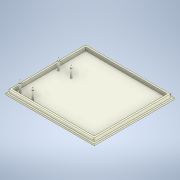
# Autodesk Inventor part: BARB_bottom
Saved by Autodesk Inventor 2022.3 (Build 263350000, 350)
## iProperties
Created: 2022-06-21
Part Number: BARB_bottom
Material: ABS Plastic
Document SubType Name: Modeling
Designer: abmos
Density: 1.06 g/cm^3
Appearance: Smooth - Ivory
Author: abmos
Autodesk Inventor part; units mm, degrees
ref_plane "YZ Plane" through (0, 0, 0) normal (1, 0, 0) x (0, 1, 0)
ref_plane "XZ Plane" through (0, 0, 0) normal (0, 1, 0) x (-1, 0, 0)
ref_plane "XY Plane" through (0, 0, 0) normal (0, 0, 1) x (1, 0, 0)
sketch "Master_XZ" plane through (0, 0, 0) normal (0, 1, 0) x (-1, 0, 0)
  line L0 (52.5, 47.5) -> (-52.5, 47.5)
  line L1 (-52.5, 47.5) -> (-52.5, -47.5)
  line L2 (-52.5, -47.5) -> (52.5, -47.5)
  line L3 (52.5, -47.5) -> (52.5, 47.5)
  line L4 (52.5, 47.5) -> (-52.5, -47.5) construction
  line L5 (-52.5, 47.5) -> (52.5, -47.5) construction
  line L6 (50.5, 45.5) -> (-50.5, 45.5)
  line L7 (-50.5, 45.5) -> (-50.5, -45.5)
  line L8 (-50.5, -45.5) -> (50.5, -45.5)
  line L9 (50.5, -45.5) -> (50.5, 45.5)
  line L10 (48.5, 43.5) -> (-48.5, 43.5)
  line L11 (-48.5, 43.5) -> (-48.5, -43.5)
  line L12 (-48.5, -43.5) -> (48.5, -43.5)
  line L13 (48.5, -43.5) -> (48.5, 43.5)
  point P0 (0, 0)
  dimension "d0" = 2
  dimension "d1" = 2
  dimension "d10" = 105
  dimension "d15" = 95
  constraints: 28 end point, 6 parallel, 3 perpendicular, 2 midpoint, 1 horizontal, 6 other
  measures "d0" distance between parallel lines of L3 L9
  measures "d1" distance between parallel lines of L9 L13
  measures "d10" distance of L0.start L0.end
  measures "d15" distance of L2.end L0.start
extrude "Floor" add sketch "Master_XZ" along normal blind 2 contours L3 L2 L1 L0 | L9 L8 L7 L6 | L13 L12 L11 L10
extrude "Walls" add sketch "Master_XZ" along normal blind 6 contours L9 L8 L7 L6
sketch "Lip_profile" plane through (0, 1, -41.5) normal (1, 0, 0) x (0, 0, -1)
  line L0 (-87, 1) -> (-87, 5) projected
  circle A0 centre (-87, 4) radius 1
  line L1 (-87, 5) -> (4, 5) projected
  line L2 (-87, 5) -> (-87, 3)
  point P0 (-41.5, -1)
  dimension "d6" = 2
  dimension "d7" = 1
  constraints: 2 end point, 1 midpoint, 1 point on line, 3 other
  measures "d7" distance from line of L1 point (-87, 4)
extrude "Lip" add sketch "Lip_profile" along normal mid plane 100
sketch "Sketch3" plane through (50, 1, -41.5) normal (1, 0, 0) x (0, 0, -1)
  line L0 (-87, 5) -> (-87, 3) projected
  line L1 (-87, 5) -> (-87, 3) projected
  arc A0 (-87, 5) -> (-87, 3) centre (-87, 4) ccw projected
  point P0 (-41.5, -1)
revolve "Lip_edge_right" add sketch "Sketch3" angle 90 about axis through (50, 6, 45.5) along (0, 1, 0)
sketch "Sketch4" plane through (-50, 1, -41.5) normal (-1, 0, 0) x (0, 0, 1)
  line L0 (87, 3) -> (87, 5) projected
  arc A0 (87, 3) -> (87, 5) centre (87, 4) ccw projected
  point P0 (41.5, -1)
revolve "Lip_edge_left" add sketch "Sketch4" angle 90 about axis through (-50, 4, 45.5) along (0, -1, 0)
pattern_circular "Circular Pattern1" count 2 over 360 about axis through (0, -10, 0) along (0, 1, 0) of "Lip", "Lip_edge_right", "Lip_edge_left"
sketch "Sketch6" plane through (0, 2, 0) normal (0, 1, 0) x (1, 0, 0)
  circle A0 centre (-44.4993, 6.9242) radius 0.6
  circle A1 centre (-29.2593, 6.9242) radius 0.6
  circle A2 centre (-29.2593, -38.7958) radius 0.6
  circle A3 centre (-44.4993, -38.7958) radius 0.6
  circle A4 centre (-29.2593, 6.9242) radius 1
  circle A5 centre (-44.4993, 6.9242) radius 1
  circle A6 centre (-44.4993, -38.7958) radius 1
  circle A7 centre (-29.2593, -38.7958) radius 1
  point P0 (0, 0)
  dimension "d18" = 1.2
  dimension "d19" = 1.2
  dimension "d20" = 1.2
  dimension "d21" = 1.2
  dimension "d22" = 45.72
  dimension "d23" = 15.24
  dimension "d26" = 0.4
  dimension "d27" = 0.4
  dimension "d28" = 0.4
  dimension "d29" = 0.4
  constraints: 8 centre point, 2 horizontal alignment, 2 vertical alignment
  measures "d18" diameter of A0
  measures "d19" diameter of A1
  measures "d20" diameter of A2
  measures "d21" diameter of A3
  measures "d22" distance of A3.centre A0.centre
  measures "d23" distance of A2.centre A3.centre
  measures "d26" radial gap between concentric circles of A1 A4
  measures "d27" radial gap between concentric circles of A0 A5
  measures "d28" radial gap between concentric circles of A3 A6
  measures "d29" radial gap between concentric circles of A2 A7
extrude "Standoff_base" add sketch "Sketch6" along normal blind 10 contours A0 | A1 | A2 | A3 | A4 | A5 | A6 | A7
sketch "Sketch8" plane through (-44.4993, 12, -6.9242) normal (0, 1, 0) x (1, 0, 0)
  circle A0 centre (0, 0) radius 1 projected
  circle A1 centre (15.24, 0) radius 1 projected
  circle A2 centre (0, -45.72) radius 1 projected
  circle A3 centre (15.24, -45.72) radius 1 projected
  circle A4 centre (0, 0) radius 0.6
  circle A5 centre (15.24, 0) radius 0.6
  circle A6 centre (0, -45.72) radius 0.6
  circle A7 centre (15.24, -45.72) radius 0.6
  point P0 (44.4993, -6.9242)
  dimension "d32" = 0.4
  dimension "d33" = 0.4
  dimension "d34" = 0.4
  dimension "d35" = 0.4
  constraints: 4 centre point
  measures "d32" radial gap between concentric circles of A0 A4
  measures "d33" radial gap between concentric circles of A1 A5
  measures "d34" radial gap between concentric circles of A2 A6
  measures "d35" radial gap between concentric circles of A3 A7
extrude "Standoff_tip" add sketch "Sketch8" along normal blind 3 draft -5 contours A4 | A5 | A6 | A7
equation "\"d27\" = d26"
equation "\"d28\" = d26"
equation "\"d29\" = d26"
equation "\"d32\" = d26"
equation "\"d33\" = d26"
equation "\"d34\" = d26"
equation "\"d35\" = d26"
